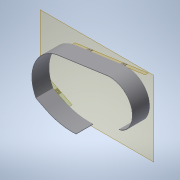
# Autodesk Inventor part: ChainGuard
Saved by Autodesk Inventor 2021 (Build 250183000, 183)
## iProperties
Created: 2020-10-28
Part Number: ChainGuard
Material: Generic
Document SubType Name: Modeling
Designer: PhotonUser
Density: 1 g/cm^3
Appearance: Default
Author: PhotonUser
Autodesk Inventor part; units mm, degrees
ref_plane "YZ Plane" through (0, 0, 0) normal (1, 0, 0) x (0, 1, 0)
ref_plane "XZ Plane" through (0, 0, 0) normal (0, 1, 0) x (-1, 0, 0)
ref_plane "XY Plane" through (0, 0, 0) normal (0, 0, 1) x (1, 0, 0)
ref_plane "Work Plane1" through (0, 0, 0) normal (0, 0, 1) x (1, 0, 0)
sketch "Sketch1" plane through (0, 0, 0) normal (0, 0, 1) x (1, 0, 0)
  line L0 (-149.3377, -84.2183) -> (-62.5438, -127.8928) projected
  arc A0 (-30.3276, 119.385) -> (-94.7251, 90.539) centre (-12.6526, -6.379) ccw projected
  line L1 (-94.7251, 90.539) -> (-158.4791, 36.5506) projected
  line L2 (267.4038, 161.2284) -> (-30.3276, 119.385) projected
  arc A1 (285.61, 2.6867) -> (293.3792, 54.1689) centre (225.4026, 38.1) ccw projected
  line L3 (293.3792, 54.1689) -> (297.7515, 151.832) projected
  line L4 (297.7015, -118.5771) -> (285.61, 2.6867) projected
  line L5 (-30.3276, 119.385) -> (187.1449, 149.9488)
  arc A2 (285.61, 2.6867) -> (187.1449, 149.9488) centre (200.8332, 52.5515) ccw
  arc A3 (240.6498, -30.0656) -> (285.61, 2.6867) centre (225.4026, 38.1) ccw
  arc A4 (-30.3276, 119.385) -> (-94.7251, 90.539) centre (-12.6526, -6.379) ccw
  line L6 (-149.3377, -84.2183) -> (-62.5438, -127.8928) projected
  line L7 (-129.8851, -94.0069) -> (-87.7502, -115.209)
  arc A5 (-94.7251, 90.539) -> (-129.8851, -94.0069) centre (1.8279, -23.4787) ccw
  arc A6 (-87.7502, -115.209) -> (48.8152, -143.0877) centre (31.9315, 122.6334) ccw
  arc A7 (-88.9193, -117.5324) -> (48.8152, -145.6938) centre (31.9315, 122.6334) ccw
  line L8 (-88.9193, -117.5324) -> (-131.786, -95.962)
  arc A8 (-96.406, 92.5238) -> (-131.786, -95.962) centre (1.8279, -23.4787) ccw
  arc A9 (-30.6896, 121.9607) -> (-96.406, 92.5238) centre (-12.6526, -6.379) ccw
  line L9 (-30.6896, 121.9607) -> (186.7829, 152.5244)
  arc A10 (287.8519, 1.3681) -> (186.7829, 152.5244) centre (200.8332, 52.5515) ccw
  arc A11 (240.6498, -32.7284) -> (287.8519, 1.3681) centre (225.4026, 38.1) ccw
  line L10 (48.8152, -145.6938) -> (48.8152, -143.0877)
  line L11 (240.6498, -32.7284) -> (240.6498, -30.0656)
  dimension "d24" = 2.601
  constraints: 20 point on circle, 12 end point, 10 centre point, 5 tangent, 2 point on line, 2 vertical, 1 collinear, 6 other
  measures "d24" radial gap between concentric circles of A5 A8
extrude "Extrusion1" add sketch "Sketch1" along normal blind 76.2 contours L0 A6 L10 A7 L8 A8 | L0 A8 L1 A5 | L1 A8 A9 L9 A10 L2 A0 | L2 A10 L3 A2 | L3 A10 A11 L4 A2 | L4 A11 L11 A3
ref_plane "Work Plane2" through (-66.6974, 114.2736, 0) normal (-0.1392, 0.9903, 0) x (-0.9903, -0.1392, 0)
sketch "Sketch2" plane through (-66.6974, 114.2736, 0) normal (-0.1392, 0.9903, 0) x (-0.9903, -0.1392, 0)
  circle A0 centre (-93.8772, -6.35) radius 2.4892 projected
  circle A1 centre (-249.4522, -6.35) radius 2.4892 projected
  line L0 (-422.3221, 0) -> (51.093, 0) projected
  line L1 (-36.7272, -12.7) -> (-337.3845, -12.7) projected
  line L2 (-36.7272, 0) -> (-256.3369, 0) projected
  line L3 (-102.8977, 0) -> (-102.8977, -12.7)
  line L4 (-83.8477, -12.7) -> (-102.8977, -12.7)
  line L5 (-83.8477, -12.7) -> (-83.8477, 0)
  circle A2 centre (-93.8772, -6.35) radius 2.4892
  line L6 (-16.5377, -12.7) -> (-16.5377, 0)
  circle A3 centre (-249.4522, -6.35) radius 2.4892
  line L7 (-354.6914, 0) -> (-256.3369, 0) projected
  line L8 (-257.8377, -12.7) -> (-238.7877, -12.7)
  line L9 (-238.7877, -12.7) -> (-238.7877, 0)
  line L10 (-257.8377, -12.7) -> (-257.8377, 0)
  line L11 (-238.7877, 0) -> (-257.8377, 0)
  line L12 (-83.8477, 0) -> (-102.8977, 0)
  line L13 (-97.2698, 0) -> (-97.2698, 76.2) projected
  point P0 (-50.1445, 0)
  point P1 (-333.3488, 0)
  dimension "d7" = 19.05
  dimension "d8" = 67.31
  dimension "d9" = 135.89
  dimension "d10" = 19.05
  constraints: 18 end point, 8 point on line, 4 vertical, 2 centre point, 2 coincident, 2 collinear, 2 concentric, 2 perpendicular, 3 other
  measures "d7" distance between parallel lines of L5 L3
  measures "d8" distance between parallel lines of L5 L6
  measures "d9" distance between parallel lines of L9 L3
  measures "d10" distance from line of L8.start L9
extrude "Extrusion2" add sketch "Sketch2" along normal blind 2.601 contours L0 L9 L1 L10 | L0 L5 L1 L3
ref_plane "Work Plane5" through (6.35, -162.56, 0) normal (-0.4495, -0.8933, 0) x (0.8933, -0.4495, 0)
sketch "Sketch5" plane through (6.35, -162.56, 0) normal (-0.4495, -0.8933, 0) x (0.8933, -0.4495, 0)
  circle A0 centre (-135.8153, -6.35) radius 2.4892 projected
  line L0 (-174.2873, 0) -> (-77.1244, 0) projected
  line L1 (-77.1244, -12.7) -> (-174.2873, -12.7) projected
  line L2 (-105.3421, 0) -> (-152.5108, 0) projected
  line L3 (-145.8483, 0) -> (-125.7823, 0)
  line L4 (-125.7823, 0) -> (-125.7823, -12.7)
  circle A1 centre (-135.8153, -6.35) radius 2.4892
  line L5 (-145.8483, 0) -> (-145.8483, -12.7)
  line L6 (-125.7823, -12.7) -> (-145.8483, -12.7)
  point P0 (-78.7426, 0)
  point P1 (-125.7823, 0)
  dimension "d25" = 10.033
  dimension "d26" = 10.033
  constraints: 8 end point, 4 point on line, 2 perpendicular, 1 centre point, 1 coincident, 1 collinear, 1 concentric
  measures "d25" distance from line of L4 A0.centre
  measures "d26" distance from line of L5 A0.centre
extrude "Extrusion5" add sketch "Sketch5" along normal blind 2.601
body "Solid1"
